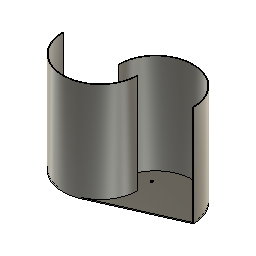
Savonius Turbine (Autodesk Fusion 360 design; units mm, degrees)
Autodesk Fusion 360 part; units mm, degrees
sketch "Turbine" plane through (0, 0, 0) normal (0, 0, 1) x (1, 0, 0) in component "Savonius Turbine"
  line L0 (10.5, 0) -> (-10.5, 0) construction
  arc A0 (74.2, 0) -> (-10.5, 0) centre (31.85, 0) ccw
  line L1 (31.85, 0) -> (74.2, 0) construction
  line L2 (31.85, 0) -> (-10.5, 0) construction
  arc A1 (-74.2, 0) -> (10.5, 0) centre (-31.85, 0) ccw
  line L3 (-31.85, 0) -> (-74.2, 0) construction
  line L4 (-31.85, 0) -> (10.5, 0) construction
  arc A2 (75, 0) -> (-11.3, 0) centre (31.85, 0) ccw
  arc A3 (-75, 0) -> (11.3, 0) centre (-31.85, 0) ccw
  line L5 (75, 0) -> (74.2, 0)
  line L6 (-75, 0) -> (-74.2, 0)
  line L7 (11.3, 0) -> (10.5, 0)
  line L8 (-10.5, 0) -> (-11.3, 0)
  line L9 (74.2, 0) -> (11.3, 0)
  line L10 (-11.3, 0) -> (-74.2, 0)
  dimension "d7" = 21
  dimension "d9" = 180
  dimension "d11" = 42.35
  dimension "d12" = 180
  dimension "d14" = 0.8
  dimension "d15" = 0.8
  constraint horizontal L0
  constraint midpoint origin L0
  constraint equal A0 A1
  constraint parallel L1 L5
  constraint parallel L3 L6
  constraint parallel L2 L7
  constraint parallel L4 L8
  constraint parallel L6 L10
  constraint collinear L0 L9
  measures "d7" distance of L0.start L0.end
  measures "d9" angle of L1 L2
  measures "d11" radius of A0
  measures "d12" angle of L3 L4
extrude "Extrude1" add sketch "Turbine" along normal blind 115.5 contours A0 A2 L5 L8 | A1 A3 L6 L7 makes body 1 at (-8.4391, -36.2471, 38.5) makes body 2 at (-4.9695, 22.4999, 38.5) in component "Savonius Turbine"
extrude "Extrude2" add sketch "Turbine" along normal blind 1.2 contours A0 A1 L7 L8 L9 L10 bodies 1 2 in component "Savonius Turbine"
sketch "Mounting Holes" plane through (0, 0, 0) normal (0, 0, 1) x (1, 0, 0) in component "Savonius Turbine"
  line L0 (-10.1657, -17.2238) -> (10.1657, 17.2238) construction
  circle A0 centre (-10.1657, -17.2238) radius 1.5
  circle A1 centre (10.1657, 17.2238) radius 1.5
  circle A2 centre (0, 0) radius 4.5
  dimension "d24" = 40
  dimension "d25" = 3
  dimension "d26" = 9
  constraint midpoint A2.centre L0
  constraint coincident L0.start A0.centre
  constraint coincident L0.end A1.centre
  constraint equal A0 A1
  constraint coincident A2.centre origin
  measures "d24" distance of L0.start L0.end
  measures "d25" diameter of A0
  measures "d26" diameter of A2
extrude "Extrude3" cut sketch "Mounting Holes" along normal through all bodies 1 in component "Savonius Turbine"
sketch "Base Reinforcement" plane through (0, 0, 0) normal (0, 0, 1) x (1, 0, 0) in component "Savonius Turbine"
  circle A0 centre (0, 0) radius 4.5
  circle A1 centre (-10.1657, -17.2238) radius 1.5
  circle A2 centre (10.1657, 17.2238) radius 1.5
  arc A3 (-75, 0) -> (11.3, 0) centre (-31.85, 0) ccw
  line L0 (-75, 0) -> (-11.3, 0)
  arc A4 (75, 0) -> (-11.3, 0) centre (31.85, 0) ccw
  line L1 (75, 0) -> (11.3, 0)
  line L2 (75, 0) -> (-14.4244, -39.475)
  line L3 (-75, 0) -> (14.4244, 39.475)
  constraint coincident A4.start L1.start
  constraint coincident A3 L2.end
  constraint tangent A3 L2
  constraint coincident A3.start L0.start
  constraint coincident A4 L3.end
  constraint tangent A4 L3
extrude "Extrude4" add sketch "Base Reinforcement" along normal blind 1.2 contours L0 A4 L3 | A3 L1 L2 bodies 1 in component "Savonius Turbine"
component "Savonius Turbine" placed x (1, 0, 0) y (0, 1, 0) z (0, 0, 1) at (0, 0, 0)
equation "Width = 150 mm" comment "Width of the turbine"
equation "AspectRatio = 0.77"
equation "OverlapPercent = 0.14" comment "How far the blades should overlap.  e.g. 0.10 would be 10%"
equation "Height = Width * AspectRatio"
equation "Overlap = OverlapPercent * Width"
equation "BladeDiameter = ( Width + Overlap ) / 2 - BladeThickness"
equation "d7 = Overlap"
equation "d11 = BladeDiameter / 2"
equation "BladeThickness = 0.8 mm"
equation "d14 = BladeThickness"
equation "d15 = BladeThickness"
equation "d19 = Height"
equation "BaseThickness = 1.2 mm"
equation "d22 = BaseThickness"
equation "d28 = BaseThickness"
named bodies: "Savonius Turbine"
